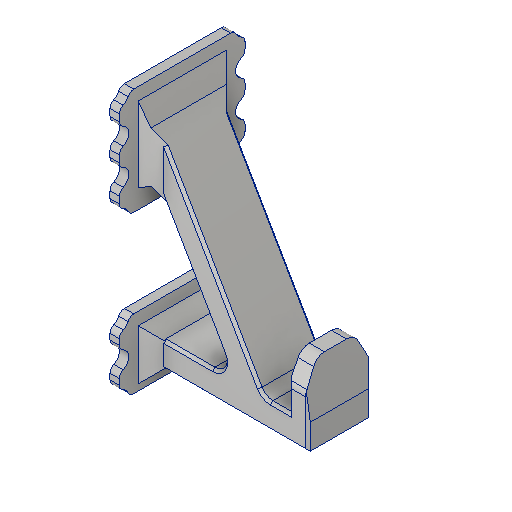
# Autodesk Inventor part: CNCM_ALU_Visual_inspection_tray_hook
Saved by Autodesk Inventor 2025 (Build 290162010, 162A)
## iProperties
Created: 2018-09-18
Part Number: CNCM_ALU_Visual_inspection_tray_hook
Material: Aluminum 6061
Document SubType Name: Modeling
Designer: Andrzej
Density: 2.7 g/cm^3
Appearance: Aluminum - Flat
Mass: 9.08107 g
Surface Area: 27.26 cm^2
Volume: 3.36336 cm^3
Author: Andrzej
Autodesk Inventor part; units mm, degrees
ref_plane "YZ Plane" through (0, 0, 0) normal (1, 0, 0) x (0, 1, 0)
ref_plane "XZ Plane" through (0, 0, 0) normal (0, 1, 0) x (-1, 0, 0)
ref_plane "XY Plane" through (0, 0, 0) normal (0, 0, 1) x (1, 0, 0)
sketch "Sketch2" plane through (0, 0, 0) normal (0, 0, 1) x (1, 0, 0)
  line L0 (-20.9816, 10.1846) -> (4.0184, 10.1846)
  line L1 (-20.9816, 14.1846) -> (4.0184, 14.1846)
  line L2 (4.0184, 14.1846) -> (4.0184, 10.1846)
  line L3 (4.0184, 14.1846) -> (4.0184, 22.1846)
  line L4 (4.0184, 22.1846) -> (1.0184, 22.1846)
  line L5 (1.0184, 22.1846) -> (1.0184, 14.1846)
  line L6 (-7.7026, 14.1846) -> (-20.9816, 37.1846)
  line L7 (-3.0838, 14.1846) -> (-20.9816, 45.1846)
  line L8 (-20.9816, 10.1846) -> (-20.9816, 14.1846)
  line L9 (-20.9816, 37.1846) -> (-20.9816, 14.1846)
  line L10 (-20.9816, 37.1846) -> (-20.9816, 45.1846)
  point P0 (0, 0)
  dimension "d0" = 25
  dimension "d1" = 3
  dimension "d2" = 4
  dimension "d3" = 4
  dimension "d4" = 35
  dimension "d5" = 60
  dimension "d14" = 8
  constraints: 22 end point, 3 perpendicular, 3 point on line, 2 collinear, 2 horizontal, 2 vertical, 1 parallel
  measures "d0" distance of L0.start L0.end
  measures "d1" distance of L3.end L4.end
  measures "d2" distance between parallel lines of L0 L1
  measures "d3" distance between parallel lines of L6 L7
  measures "d4" distance of L0.start L7.end
  measures "d5" angle of L1 L6
  measures "d14" distance of L1.end L3.end
extrude "Extrusion1" add sketch "Sketch2" along normal blind 10 contours L8 L1 L2 L0 | L1 L5 L4 L3 | L6 L10 L7 L1
sketch "Sketch3" plane through (-20.9816, 37.1846, 0) normal (-1, 0, 0) x (0, 0, 1)
  line L0 (-5, 15) -> (15, 15)
  line L1 (15, 15) -> (15, -30)
  line L2 (15, -30) -> (-5, -30)
  line L3 (-5, -30) -> (-5, 15)
  line L4 (0, 8) -> (0, 0) projected
  line L5 (0, 0) -> (10, 0) projected
  line L6 (10, 8) -> (10, 0) projected
  line L7 (0, 8) -> (10, 8) projected
  line L8 (0, -23) -> (0, -27) projected
  line L9 (0, -27) -> (10, -27) projected
  line L10 (10, -23) -> (10, -27) projected
  line L11 (0, -23) -> (10, -23) projected
  line L12 (-5, -19) -> (15, -19)
  line L13 (-5, 12) -> (15, 12)
  line L14 (-5, -5) -> (15, -5)
  circle A0 centre (-5, 12) radius 1.5
  circle A1 centre (15, 12) radius 1.5
  circle A2 centre (-5, -19) radius 1.5
  circle A3 centre (-5, -30) radius 1.5
  circle A4 centre (15, -30) radius 1.5
  circle A5 centre (15, -19) radius 1.5
  circle A6 centre (-5, -24.5) radius 1.5
  circle A7 centre (15, -24.5) radius 1.5
  circle A8 centre (-5, 6.3333) radius 1.5
  circle A9 centre (-5, 0.6667) radius 1.5
  circle A10 centre (-5, -5) radius 1.5
  circle A11 centre (15, 6.3333) radius 1.5
  circle A12 centre (15, 0.6667) radius 1.5
  circle A13 centre (15, -5) radius 1.5
  point P0 (0, -37.1846)
  dimension "d15" = 20
  dimension "d16" = 45
  dimension "d17" = 3
  dimension "d18" = 10
  dimension "d19" = 5
  dimension "d20" = 4
  dimension "d21" = 5
  dimension "d22" = 4
  dimension "d25" = 3
  dimension "d28" = 3
  dimension "d29" = 3
  dimension "d30" = 3
  dimension "d31" = 3
  dimension "d32" = 3
  dimension "d33" = 3
  dimension "d34" = 3
  dimension "d35" = 11
  dimension "d36" = 5.5
  dimension "d37" = 17
  dimension "d40" = 5.6667
  dimension "d47" = 5.6667
  constraints: 14 centre point, 14 end point, 12 coincident, 8 point on line, 3 perpendicular, 2 horizontal, 2 parallel, 2 vertical, 1 horizontal alignment, 18 other
  measures "d15" distance of L1.end L2.end
  measures "d16" distance of L0.end L1.end
  measures "d17" distance between parallel lines of L2 L9
  measures "d18" distance between parallel lines of L10 L8
  measures "d19" distance between parallel lines of L3 L8
  measures "d20" distance between parallel lines of L12 L11
  measures "d21" distance between parallel lines of L14 L5
  measures "d22" distance between parallel lines of L7 L13
  measures "d25" diameter of A0
  measures "d28" diameter of A1
  measures "d29" diameter of A2
  measures "d30" diameter of A3
  measures "d31" diameter of A4
  measures "d32" diameter of A5
  measures "d33" diameter of A6
  measures "d34" diameter of A7
  measures "d35" distance between parallel lines of L2 L12
  measures "d36" distance from line of L12 A6.centre
  measures "d37" distance between parallel lines of L14 L13
  measures "d40" distance of A0.centre A8.centre
  measures "d47" distance of A1.centre A11.centre
extrude "Extrusion2" add sketch "Sketch3" along normal blind 1.5 contours L13 A0 L3 | L13 A1 L1 A11 A12 A13 L14 A10 L3 A9 A8 A0 | L1 A1 L13 | A8 L3 | L1 A11 | A9 L3 | L1 A12 | A10 L14 L3 | L1 L14 A13 | L12 A2 L3 | L12 A5 L1 A7 A4 L2 A3 L3 A6 A2 | L12 L1 A5 | A6 L3 | L1 A7 | A3 L2 L3 | L1 L2 A4 | L7 L6 L5 L4 | L11 L10 L9 L8 picked at (-4.6718, 11.0621) picked at (14.0125, 11.8887) picked at (-4.2378, 6.0073) picked at (14.3164, 6.7503) picked at (-4.577, 1.0702) picked at (14.3164, 1.0837) picked at (-4.8887, -4.0125) picked at (14.0125, -4.8887) picked at (-4.6718, -19.9379) picked at (14.8887, -19.9875) picked at (-4.8887, -24.0125) picked at (14.0246, -24.1475) picked at (-4.0621, -29.6718) picked at (14.0125, -29.8887)
extrude "Extrusion3" cut sketch "Sketch3" along normal blind 2 contours A0 L13 L3 | L3 A0 | A1 L1 | L1 L13 A1 | L13 A0 L3 | L1 A1 L13 | A8 L3 | L3 A8 | A11 L1 | L1 A11 | A9 L3 | L3 A9 | A12 L1 | L1 A12 | A10 L14 L3 | L3 A10 | L14 A10 L3 | A13 L1 | L1 L14 A13 | L14 L1 A13 | A2 L12 L3 | L3 A2 | L12 A2 L3 | A5 L1 | L1 L12 A5 | L12 L1 A5 | A6 L3 | L3 A6 | A7 L1 | L1 A7 | A3 L2 L3 | L3 L2 A3 | A4 L2 L1 | L1 L2 A4
chamfer "Chamfer3" distance 2 angle 45 8 edges at (-20.9816, 41.1846, 0) (-20.9816, 45.1846, 5) (-20.9816, 41.1846, 10) (-20.9816, 37.1846, 5) (-20.9816, 12.1846, 10) (-20.9816, 14.1846, 5) (-20.9816, 10.1846, 5) (-20.9816, 12.1846, 0)
fillet "Fillet1" radius 2 2 edges at (-3.0838, 14.1846, 5) (-7.7026, 14.1846, 5)
chamfer "Chamfer4" distance 0.4 angle 45 16 edges at (-11.3214, 28.4526, 10) (-2.9291, 14.4526, 10) (-0.4553, 14.1846, 10) (-14.2081, 25.4526, 10) (-15.0741, 14.1846, 10) (-11.3214, 28.4526, 0) (-2.9291, 14.4526, 0) (-0.4553, 14.1846, 0) (-14.2081, 25.4526, 0) (-15.0741, 14.1846, 0) (1.0184, 18.1846, 10) (4.0184, 16.1846, 10) (4.0184, 16.1846, 0) (-7.4816, 10.1846, 10) (-7.4816, 10.1846, 0) (1.0184, 18.1846, 0)
chamfer "Chamfer5" distance 0.6 distance2 8 1 edges at (4.0184, 22.1846, 5) measured on face at (3.0184, 22.1846, 6.5333)
chamfer "Chamfer6" distance 2 distance2 4 1 edges at (2.4184, 22.1846, 0) measured on face at (2.6184, 22.1846, 3.4667)
chamfer "Chamfer7" distance 2 distance2 4 1 edges at (2.4184, 22.1846, 10) measured on face at (2.6184, 22.1846, 7.2)
fillet "Fillet2" radius 2 4 edges at (2.2184, 22.1846, 2) (2.5184, 18.1846, 0) (2.2184, 22.1846, 8) (2.5184, 18.1846, 10)
fillet "Fillet3" radius 1 28 edges at (-21.7316, 49.1846, -3.5) (-21.7316, 47.6846, -5) (-21.7316, 45.018, -5) (-21.7316, 42.018, -5) (-21.7316, 39.3513, -5) (-21.7316, 36.3513, -5) (-21.7316, 33.6846, -5) (-21.7316, 32.1846, -3.5) (-21.7316, 49.1846, 13.5) (-21.7316, 47.6846, 15) (-21.7316, 42.018, 15) (-21.7316, 45.018, 15) (-21.7316, 36.3513, 15) (-21.7316, 39.3513, 15) (-21.7316, 33.6846, 15) (-21.7316, 32.1846, 13.5) (-21.7316, 18.1846, 13.5) (-21.7316, 16.6846, 15) (-21.7316, 11.1846, 15) (-21.7316, 14.1846, 15) (-21.7316, 8.6846, 15) (-21.7316, 7.1846, 13.5) (-21.7316, 7.1846, -3.5) (-21.7316, 8.6846, -5) (-21.7316, 14.1846, -5) (-21.7316, 11.1846, -5) (-21.7316, 16.6846, -5) (-21.7316, 18.1846, -3.5)
equation "\"d3\" = d2"
equation "\"d36\" = 0.5 * d35"
body "Solid1"
